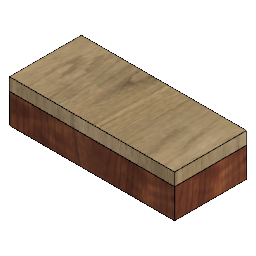
TeaBox v16 (Autodesk Fusion 360 design; units mm, degrees)
Autodesk Fusion 360 part; units mm, degrees
note: some values were not read from the file. Chosen so that the rebuilt part matches the saved one: which face or edge a step refers to. Set by a fixed rule: which sketch regions a step uses.
sketch "Sketch1" plane through (0, 0, 0) normal (0, 0, 1) x (1, 0, 0)
  line L0 (0, 0) -> (69.85, 0)
  line L1 (69.85, 0) -> (69.85, 82.55)
  line L2 (69.85, 82.55) -> (0, 82.55)
  line L3 (0, 82.55) -> (0, 0)
  line L4 (146.05, 0) -> (146.05, 82.55)
  line L5 (76.2, 82.55) -> (76.2, 0)
  line L6 (146.05, 82.55) -> (76.2, 82.55)
  line L7 (76.2, 0) -> (146.05, 0)
  line L8 (222.25, 0) -> (222.25, 82.55)
  line L9 (152.4, 82.55) -> (152.4, 0)
  line L10 (222.25, 82.55) -> (152.4, 82.55)
  line L11 (152.4, 0) -> (222.25, 0)
  line L12 (-12.7, -12.7) -> (234.95, -12.7)
  line L13 (234.95, -12.7) -> (234.95, 95.25)
  line L14 (234.95, 95.25) -> (-12.7, 95.25)
  line L15 (-12.7, 95.25) -> (-12.7, -12.7)
  dimension "d1" = 82.55
  dimension "d2" = 69.85
  dimension "d7" = 82.55
  dimension "d8" = 69.85
  dimension "d9" = 82.55
  dimension "d10" = 69.85
  dimension "d13" = 6.35
  dimension "d14" = 6.35
  dimension "d16" = 12.7
  dimension "d17" = 12.7
  dimension "d53" = 12.7
  measures "d1" distance of L0.start
  measures "d2" distance of L0.start
  measures "d9" distance of L0.start
  measures "d13" distance of L1 L5
  measures "d14" distance of L4 L9
  measures "d16" distance of L2 L14
  measures "d17" distance of L3 L15
  measures "d53" distance of L8 L13
extrude "Extrude1" add sketch "Sketch1" against normal blind 12.7 contours L0 L1 L2 L3 | L4 L5 L6 L7 | L8 L9 L10 L11 | L12 L13 L14 L15 makes body 1
extrude "Extrude2" add sketch "Sketch1" along normal blind 31.75 bodies 1
fillet "Fillet1" radius 3.175 12 edges at (0, 0, 15.875) (69.85, 0, 15.875) (69.85, 82.55, 15.875) (0, 82.55, 15.875) (146.05, 0, 15.875) (146.05, 82.55, 15.875) (76.2, 82.55, 15.875) (76.2, 0, 15.875) (222.25, 0, 15.875) (222.25, 82.55, 15.875) (152.4, 82.55, 15.875) (152.4, 0, 15.875) on bodies 1
copy_body "Body->Comp1" bodies 1 removing the originals makes body 2 in component "Component"
sketch "Sketch3" plane through (0, 0, 31.75) normal (0, 0, 1) x (-1, 0, 0)
  line L0 (12.7, -95.25) -> (12.7, 12.7)
  line L1 (12.7, 12.7) -> (-234.95, 12.7)
  line L2 (-234.95, 12.7) -> (-234.95, -95.25)
  line L3 (-234.95, -95.25) -> (12.7, -95.25)
  line L4 (-234.95, -95.25) -> (12.7, -95.25)
  line L5 (6.35, -88.9) -> (-304.8, -88.9)
  line L6 (12.7, -95.25) -> (12.7, 12.7)
  line L7 (6.35, 6.35) -> (6.35, -88.9)
  line L8 (-304.8, 6.35) -> (6.35, 6.35)
  line L9 (12.7, 12.7) -> (-234.95, 12.7)
  line L10 (-304.8, -88.9) -> (-304.8, 6.35)
  line L11 (-234.95, 12.7) -> (-234.95, -95.25)
  arc A0 through (-219.075, 0, -31.75) (-221.3201, -0.9299, -31.75) (-222.25, -3.175, -31.75)
  line L12 (-222.25, -3.175, -31.75) -> (-222.25, -79.375, -31.75)
  arc A1 through (-222.25, -79.375, -31.75) (-221.3201, -81.6201, -31.75) (-219.075, -82.55, -31.75)
  line L13 (-219.075, -82.55, -31.75) -> (-155.575, -82.55, -31.75)
  arc A2 through (-155.575, -82.55, -31.75) (-153.3299, -81.6201, -31.75) (-152.4, -79.375, -31.75)
  line L14 (-152.4, -79.375, -31.75) -> (-152.4, -3.175, -31.75)
  arc A3 through (-152.4, -3.175, -31.75) (-153.3299, -0.9299, -31.75) (-155.575, 0, -31.75)
  line L15 (-155.575, 0, -31.75) -> (-219.075, 0, -31.75)
  arc A4 through (-79.375, -82.55, -31.75) (-77.1299, -81.6201, -31.75) (-76.2, -79.375, -31.75)
  line L16 (-76.2, -79.375, -31.75) -> (-76.2, -3.175, -31.75)
  arc A5 through (-76.2, -3.175, -31.75) (-77.1299, -0.9299, -31.75) (-79.375, 0, -31.75)
  line L17 (-79.375, 0, -31.75) -> (-142.875, 0, -31.75)
  arc A6 through (-142.875, 0, -31.75) (-145.1201, -0.9299, -31.75) (-146.05, -3.175, -31.75)
  line L18 (-146.05, -3.175, -31.75) -> (-146.05, -79.375, -31.75)
  arc A7 through (-146.05, -79.375, -31.75) (-145.1201, -81.6201, -31.75) (-142.875, -82.55, -31.75)
  line L19 (-142.875, -82.55, -31.75) -> (-79.375, -82.55, -31.75)
  arc A8 through (0, -3.175, -31.75) (-0.9299, -0.9299, -31.75) (-3.175, 0, -31.75)
  line L20 (-3.175, 0, -31.75) -> (-66.675, 0, -31.75)
  arc A9 through (-66.675, 0, -31.75) (-68.9201, -0.9299, -31.75) (-69.85, -3.175, -31.75)
  line L21 (-69.85, -3.175, -31.75) -> (-69.85, -79.375, -31.75)
  arc A10 through (-69.85, -79.375, -31.75) (-68.9201, -81.6201, -31.75) (-66.675, -82.55, -31.75)
  line L22 (-66.675, -82.55, -31.75) -> (-3.175, -82.55, -31.75)
  arc A11 through (-3.175, -82.55, -31.75) (-0.9299, -81.6201, -31.75) (0, -79.375, -31.75)
  line L23 (0, -79.375, -31.75) -> (0, -3.175, -31.75)
  line L24 (-219.075, 0) -> (-155.575, 0)
  arc A12 (-152.4, -3.175) -> (-155.575, 0) centre (-155.575, -3.175) ccw
  line L25 (-152.4, -3.175) -> (-152.4, -79.375)
  arc A13 (-155.575, -82.55) -> (-152.4, -79.375) centre (-155.575, -79.375) ccw
  line L26 (-155.575, -82.55) -> (-219.075, -82.55)
  arc A14 (-222.25, -79.375) -> (-219.075, -82.55) centre (-219.075, -79.375) ccw
  line L27 (-222.25, -79.375) -> (-222.25, -3.175)
  arc A15 (-219.075, 0) -> (-222.25, -3.175) centre (-219.075, -3.175) ccw
  line L28 (-142.875, 0) -> (-79.375, 0)
  arc A16 (-76.2, -3.175) -> (-79.375, 0) centre (-79.375, -3.175) ccw
  line L29 (-76.2, -3.175) -> (-76.2, -79.375)
  arc A17 (-79.375, -82.55) -> (-76.2, -79.375) centre (-79.375, -79.375) ccw
  line L30 (-79.375, -82.55) -> (-142.875, -82.55)
  arc A18 (-146.05, -79.375) -> (-142.875, -82.55) centre (-142.875, -79.375) ccw
  line L31 (-146.05, -79.375) -> (-146.05, -3.175)
  arc A19 (-142.875, 0) -> (-146.05, -3.175) centre (-142.875, -3.175) ccw
  line L32 (0, -3.175) -> (0, -79.375)
  arc A20 (-3.175, -82.55) -> (0, -79.375) centre (-3.175, -79.375) ccw
  line L33 (-3.175, -82.55) -> (-66.675, -82.55)
  arc A21 (-69.85, -79.375) -> (-66.675, -82.55) centre (-66.675, -79.375) ccw
  line L34 (-69.85, -79.375) -> (-69.85, -3.175)
  arc A22 (-66.675, 0) -> (-69.85, -3.175) centre (-66.675, -3.175) ccw
  line L35 (-66.675, 0) -> (-3.175, 0)
  arc A23 (0, -3.175) -> (-3.175, 0) centre (-3.175, -3.175) ccw
  arc A24 through (-79.375, -82.55, -31.75) (-77.1299, -81.6201, -31.75) (-76.2, -79.375, -31.75)
  line L36 (-76.2, -79.375, -31.75) -> (-76.2, -3.175, -31.75)
  arc A25 through (-76.2, -3.175, -31.75) (-77.1299, -0.9299, -31.75) (-79.375, 0, -31.75)
  line L37 (-79.375, 0, -31.75) -> (-142.875, 0, -31.75)
  arc A26 through (-142.875, 0, -31.75) (-145.1201, -0.9299, -31.75) (-146.05, -3.175, -31.75)
  line L38 (-146.05, -3.175, -31.75) -> (-146.05, -79.375, -31.75)
  arc A27 through (-146.05, -79.375, -31.75) (-145.1201, -81.6201, -31.75) (-142.875, -82.55, -31.75)
  line L39 (-142.875, -82.55, -31.75) -> (-79.375, -82.55, -31.75)
  arc A28 through (-219.075, 0, -31.75) (-221.3201, -0.9299, -31.75) (-222.25, -3.175, -31.75)
  line L40 (-222.25, -3.175, -31.75) -> (-222.25, -79.375, -31.75)
  arc A29 through (-222.25, -79.375, -31.75) (-221.3201, -81.6201, -31.75) (-219.075, -82.55, -31.75)
  line L41 (-219.075, -82.55, -31.75) -> (-155.575, -82.55, -31.75)
  arc A30 through (-155.575, -82.55, -31.75) (-153.3299, -81.6201, -31.75) (-152.4, -79.375, -31.75)
  line L42 (-152.4, -79.375, -31.75) -> (-152.4, -3.175, -31.75)
  arc A31 through (-152.4, -3.175, -31.75) (-153.3299, -0.9299, -31.75) (-155.575, 0, -31.75)
  line L43 (-155.575, 0, -31.75) -> (-219.075, 0, -31.75)
  arc A32 through (0, -3.175, -31.75) (-0.9299, -0.9299, -31.75) (-3.175, 0, -31.75)
  line L44 (-3.175, 0, -31.75) -> (-66.675, 0, -31.75)
  arc A33 through (-66.675, 0, -31.75) (-68.9201, -0.9299, -31.75) (-69.85, -3.175, -31.75)
  line L45 (-69.85, -3.175, -31.75) -> (-69.85, -79.375, -31.75)
  arc A34 through (-69.85, -79.375, -31.75) (-68.9201, -81.6201, -31.75) (-66.675, -82.55, -31.75)
  line L46 (-66.675, -82.55, -31.75) -> (-3.175, -82.55, -31.75)
  arc A35 through (-3.175, -82.55, -31.75) (-0.9299, -81.6201, -31.75) (0, -79.375, -31.75)
  line L47 (0, -79.375, -31.75) -> (0, -3.175, -31.75)
extrude "Extrude1'" add sketch "Sketch3" along normal blind 19.05 separate body contours L0 L1 L2 L3 L4 L5 L6 L7 L8 L9 L11 | L2 L5 L7 L8 L11 | L24 A12 L25 A13 L26 A14 L27 A15 | L28 A16 L29 A17 L30 A18 L31 A19 | L32 A20 L33 A21 L34 A22 L35 A23 makes body 3 in component "Component'"
sketch "Sketch5" plane through (0, 0, 31.75) normal (0, 0, -1) x (1, 0, 0)
  line L0 (234.95, -95.25) -> (234.95, 12.7)
  line L1 (234.95, 12.7) -> (-12.7, 12.7)
  line L2 (-12.7, 12.7) -> (-12.7, -95.25)
  line L3 (-12.7, -95.25) -> (234.95, -95.25)
  line L4 (234.95, 12.7) -> (234.95, -95.25)
  line L5 (234.95, -95.25) -> (-12.7, -95.25)
  line L6 (-12.7, -95.25) -> (-12.7, 12.7)
  line L7 (-12.7, 12.7) -> (234.95, 12.7)
  line L8 (0, -82.55) -> (222.25, -82.55)
  line L9 (222.25, -82.55) -> (222.25, 0)
  line L10 (222.25, 0) -> (0, 0)
  line L11 (0, 0) -> (0, -82.55)
  dimension "d50" = 12.7
  measures "d50" distance of L3
extrude "Extrude6" cut sketch "Sketch5" against normal blind 12.7 contours L8 L9 L10 L11 bodies 3 in component "Component'"
component "Component'" placed x (1, 0, 0) y (0, 1, 0) z (0, 0, 1) at (0, 0, 0)
component "Component" placed x (1, 0, 0) y (0, 1, 0) z (0, 0, 1) at (0, 0, 0)
